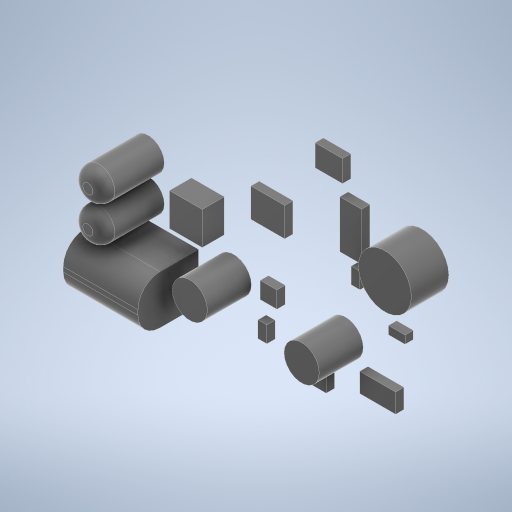
# Autodesk Inventor part: Part2
Saved by Autodesk Inventor 2023 (Build 270158000, 158)
## iProperties
Created: 2024-10-12
Part Number: Part2
Material: PBT Plastic
Document SubType Name: Modeling
Designer: noname
Density: 1.31 g/cm^3
Appearance: Smooth - Black
Author: noname
Autodesk Inventor part; units mm, degrees
ref_plane "YZ Plane" through (0, 0, 0) normal (1, 0, 0) x (0, 1, 0)
ref_plane "XZ Plane" through (0, 0, 0) normal (0, 1, 0) x (-1, 0, 0)
ref_plane "XY Plane" through (0, 0, 0) normal (0, 0, 1) x (1, 0, 0)
sketch "Sketch1" plane through (0, 0, 0) normal (0, 0, 1) x (1, 0, 0)
  line L0 (-0.340855, -0.519684) -> (-6.486214, -0.519684)
  line L1 (-6.486214, -0.519684) -> (-6.486214, 4.735944)
  line L2 (-6.486214, 4.735944) -> (-0.340855, 4.735944)
  line L3 (-0.340855, 4.735944) -> (-0.340855, -0.519684)
  line L4 (7.200496, -21.069022) -> (3.194116, -21.069022)
  line L5 (3.194116, -21.069022) -> (3.194116, -17.121995)
  line L6 (3.194116, -17.121995) -> (7.200496, -17.121995)
  line L7 (7.200496, -17.121995) -> (7.200496, -21.069022)
  line L8 (19.842852, -18.071656) -> (13.313936, -18.071656)
  line L9 (13.313936, -18.071656) -> (13.313936, -14.569783)
  line L10 (13.313936, -14.569783) -> (19.842852, -14.569783)
  line L11 (19.842852, -14.569783) -> (19.842852, -18.071656)
  line L12 (13.640382, 2.464751) -> (9.693355, 2.464751)
  line L13 (9.693355, 2.464751) -> (9.693355, 11.130403)
  line L14 (9.693355, 11.130403) -> (13.640382, 11.130403)
  line L15 (13.640382, 11.130403) -> (13.640382, 2.464751)
  line L16 (10.168186, 13.4452) -> (5.197306, 13.4452)
  line L17 (5.197306, 13.4452) -> (5.197306, 17.392226)
  line L18 (5.197306, 17.392226) -> (10.168186, 17.392226)
  line L19 (10.168186, 17.392226) -> (10.168186, 13.4452)
  line L20 (11.751959, -1.6996) -> (13.347204, -1.6996)
  line L21 (13.347204, -1.6996) -> (13.347204, 1.218509)
  line L22 (13.347204, 1.218509) -> (11.751959, 1.218509)
  line L23 (11.751959, 1.218509) -> (11.751959, -1.6996)
  line L24 (21.547875, -6.190323) -> (18.530226, -6.190323)
  line L25 (18.530226, -6.190323) -> (18.530226, -4.741215)
  line L26 (18.530226, -4.741215) -> (21.547875, -4.741215)
  line L27 (21.547875, -4.741215) -> (21.547875, -6.190323)
  line L28 (-1.753422, -12.313538) -> (-4.791311, -12.313538)
  line L29 (-4.791311, -12.313538) -> (-4.791311, -9.292684)
  line L30 (-4.791311, -9.292684) -> (-1.753422, -9.292684)
  line L31 (-1.753422, -9.292684) -> (-1.753422, -12.313538)
  line L32 (-3.585641, -18.67975) -> (-5.213094, -18.67975)
  line L33 (-5.213094, -18.67975) -> (-5.213094, -15.724234)
  line L34 (-5.213094, -15.724234) -> (-3.585641, -15.724234)
  line L35 (-3.585641, -15.724234) -> (-3.585641, -18.67975)
  line L36 (-17.54718, -20.399792) -> (-31.142779, -20.399792)
  line L37 (-31.142779, -20.399792) -> (-31.142779, -11.536708)
  line L38 (-31.142779, -11.536708) -> (-17.54718, -11.536708)
  line L39 (-17.54718, -11.536708) -> (-17.54718, -20.399792)
  line L40 (-12.839976, -6.88519) -> (-18.805889, -6.88519)
  line L41 (-18.805889, -6.88519) -> (-18.805889, -0.8921)
  line L42 (-18.805889, -0.8921) -> (-12.839976, -0.8921)
  line L43 (-12.839976, -0.8921) -> (-12.839976, -6.88519)
  line L44 (25, 22.5) -> (-27.5, 22.5)
  line L45 (-30, 2.5) -> (-30, -20)
  circle A0 centre (-26.667866, -1.031426) radius 2.914638
  circle A1 centre (-26.667866, -7.509644) radius 2.914638
  circle A2 centre (23.182784, 7.204764) radius 4.825261
  circle A3 centre (-11.114227, -12.313538) radius 3.201373
  circle A4 centre (9.236423, -12.010573) radius 3.201373
  circle A5 centre (-4, 17.5) radius 2.5
  circle A6 centre (-4, 17.5) radius 2.5
  circle A7 centre (-4, 17.5) radius 2.82145
  circle A8 centre (-4, 17.5) radius 2.82145
  circle A9 centre (-4, 17.5) radius 2.82145
  point P0 (0, 0)
  constraints: 88 end point, 22 parallel, 11 horizontal, 11 perpendicular, 9 centre point, 4 coincident, 4 equal radius, 1 vertical alignment
extrude "Extrusion2" add sketch "Sketch1" along normal blind 1.5 contours L0 L1 L2 L3 | L4 L5 L6 L7 | L8 L9 L10 L11 | L12 L13 L14 L15 | L16 L17 L18 L19 | L23 L22 L21 L20 | L24 L25 L26 L27 | L28 L29 L30 L31 | L32 L33 L34 L35 | L36 L37 L38 L39 | L40 L41 L42 L43 | A0 | A1 | A2 | A3 | A4
sketch "Sketch4" plane through (0, 0, 1.5) normal (0, 0, 1) x (1, 0, 0)
  circle A0 centre (23.182784, 7.204764) radius 4.825261
  circle A1 centre (9.236423, -12.010573) radius 3.201373
  circle A2 centre (-11.114227, -12.313538) radius 3.201373
  circle A3 centre (-26.667866, -7.509644) radius 2.914638
  circle A4 centre (-26.667866, -1.031426) radius 2.914638
  line L0 (-31.142779, -20.399792) -> (-17.54718, -20.399792)
  line L1 (-17.54718, -20.399792) -> (-17.54718, -11.536708)
  line L2 (-17.54718, -11.536708) -> (-31.142779, -11.536708)
  line L3 (-31.142779, -11.536708) -> (-31.142779, -20.399792)
  line L4 (-12.839976, -0.8921) -> (-18.805889, -0.8921)
  line L5 (-18.805889, -0.8921) -> (-18.805889, -6.88519)
  line L6 (-18.805889, -6.88519) -> (-12.839976, -6.88519)
  line L7 (-12.839976, -6.88519) -> (-12.839976, -0.8921)
  point P0 (0, 0)
extrude "Extrusion3" add sketch "Sketch4" along normal blind 2.5
sketch "Sketch5" plane through (23.182784, 7.204764, 4) normal (0, 0, 1) x (1, 0, 0)
  circle A0 centre (0, 0) radius 4.825261
  circle A1 centre (-13.946361, -19.215338) radius 3.201373
  circle A2 centre (-34.29701, -19.518302) radius 3.201373
  circle A3 centre (-49.85065, -8.23619) radius 2.914638
  circle A4 centre (-49.85065, -14.714408) radius 2.914638
  line L0 (-40.729964, -27.604557) -> (-40.729964, -18.741472)
  line L1 (-40.729964, -18.741472) -> (-54.325562, -18.741472)
  line L2 (-54.325562, -18.741472) -> (-54.325562, -27.604557)
  line L3 (-54.325562, -27.604557) -> (-40.729964, -27.604557)
  point P0 (-23.182784, -7.204764)
extrude "Extrusion4" add sketch "Sketch5" along normal blind 2.8
sketch "Sketch6" plane through (-11.114227, -12.313538, 6.8) normal (0, 0, 1) x (1, 0, 0)
  circle A0 centre (20.35065, 0.302965) radius 3.201373
  circle A1 centre (0, 0) radius 3.201373
  circle A2 centre (-15.553639, 4.803894) radius 2.914638
  circle A3 centre (-15.553639, 11.282112) radius 2.914638
  line L0 (-6.432953, 0.77683) -> (-20.028552, 0.77683)
  line L1 (-20.028552, 0.77683) -> (-20.028552, -8.086254)
  line L2 (-20.028552, -8.086254) -> (-6.432953, -8.086254)
  line L3 (-6.432953, -8.086254) -> (-6.432953, 0.77683)
  point P0 (11.114227, 12.313538)
extrude "Extrusion5" add sketch "Sketch6" along normal blind 1.2
sketch "Sketch7" plane through (-11.114227, -12.313538, 8) normal (0, 0, 1) x (1, 0, 0)
  line L0 (-20.028552, 0.77683) -> (-20.028552, -8.086254)
  line L1 (-20.028552, -8.086254) -> (-6.432953, -8.086254)
  line L2 (-6.432953, -8.086254) -> (-6.432953, 0.77683)
  line L3 (-6.432953, 0.77683) -> (-20.028552, 0.77683)
  circle A0 centre (-15.553639, 4.803894) radius 2.914638
  circle A1 centre (-15.553639, 11.282112) radius 2.914638
  point P0 (11.114227, 12.313538)
extrude "Extrusion6" add sketch "Sketch7" along normal blind 3
fillet "Fillet1" radius 4 2 edges at (-24.345, -11.5367, 11) (-24.345, -20.3998, 11)
fillet "Fillet2" radius 2 2 edges at (-29.5825, -1.0314, 11) (-29.5825, -7.5096, 11)
body "Solid2"
